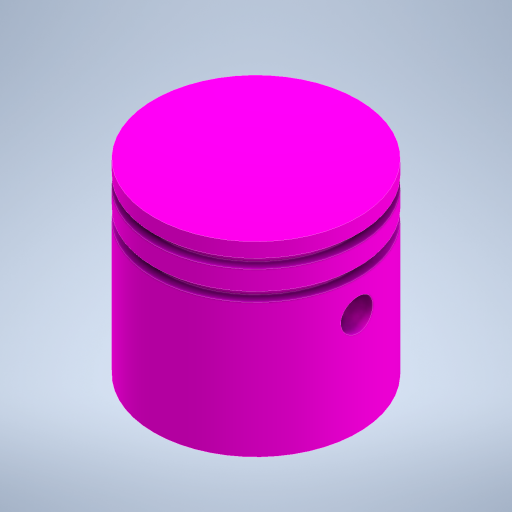
# Autodesk Inventor part: Piston_head
Saved by Autodesk Inventor 2024 (Build 280153000, 153)
## iProperties
Created: 2023-11-02
Part Number: Piston_head
Material: Ocel
Document SubType Name: Modeling
Designer: zak
Density: 7.85 g/cm^3
Appearance: Purpurová
Author: zak
Autodesk Inventor part; units mm, degrees
ref_plane "XZ Plane" through (0, 0, 0) normal (0, 1, 0) x (-1, 0, 0)
ref_plane "XY Plane" through (0, 0, 0) normal (0, 0, 1) x (1, 0, 0)
sketch "Náčrt3" plane through (0, 0, 0) normal (1, 0, 0) x (0, 1, 0)
  line L0 (0, 0) -> (0, 16)
  line L1 (0, 16) -> (21, 16)
  line L2 (21, 16) -> (21, 14.5)
  line L3 (21, 14.5) -> (22.5, 14.5)
  line L4 (22.5, 14.5) -> (22.5, 16)
  line L5 (22.5, 16) -> (25.5, 16)
  line L6 (25.5, 16) -> (25.5, 14.5)
  line L7 (25.5, 14.5) -> (27, 14.5)
  line L8 (27, 14.5) -> (27, 16)
  line L9 (27, 16) -> (29.2548, 16)
  line L10 (32, 0) -> (0, 0)
  arc A0 (32, 0) -> (29.2548, 16) centre (-16, 0) ccw
  dimension "d4" = 16
  dimension "d5" = 21
  dimension "d6" = 3
  dimension "d7" = 1.5
  dimension "d8" = 1.5
  dimension "d9" = 14.5
  dimension "d12" = 96
  dimension "d13" = 32
  constraints: 22 end point, 8 perpendicular, 2 collinear, 2 point on circle, 2 point on line, 1 centre point, 1 parallel, 1 vertical
  measures "d4" distance between parallel lines of L10 L1
  measures "d5" distance between parallel lines of L2 L0
  measures "d6" distance between parallel lines of L6 L4
  measures "d7" distance of L2.end L3.end
  measures "d8" distance of L6.end L7.end
  measures "d9" distance between parallel lines of L10 L3
  measures "d12" diameter of A0
  measures "d13" distance of L0.start L10.start
revolve "Rotace1" add sketch "Náčrt3" angle 360 about axis through (0, 32, 0) along (0, -1, 0)
sketch "Náčrt4" plane through (0, 0, 0) normal (1, 0, 0) x (0, 1, 0)
  line L0 (0, 16) -> (0, -16) projected
  line L1 (0, 13) -> (10, 13)
  line L2 (10, 13) -> (10, 10)
  line L3 (20.5263, 0) -> (0, 0)
  line L4 (10, 10) -> (24, 10)
  line L5 (24, 10) -> (24, 0)
  line L6 (24, 0) -> (20.5263, 0)
  line L7 (-6.4, 0) -> (38.4, 0) projected
  dimension "d14" = 10
  dimension "d15" = 13
  dimension "d16" = 10
  dimension "d17" = 24
  constraints: 12 end point, 3 perpendicular, 2 horizontal, 1 point on line, 1 vertical
  measures "d14" distance between parallel lines of L6 L4
  measures "d15" distance between parallel lines of L3 L1
  measures "d16" distance between parallel lines of L0 L2
  measures "d17" distance between parallel lines of L0 L5
revolve "Rotace2" cut sketch "Náčrt4" angle 360 about axis through (0, -10, 0) along (0, 1, 0)
fillet "Zaoblení1" radius 2 2 edges at (0, 10, -13) (0, 24, -10)
ref_plane "Pracovní rovina1" through (16, 0, 0) normal (1, 0, 0) x (0, 1, 0)
sketch "Náčrt5" plane through (16, 0, 0) normal (1, 0, 0) x (0, 1, 0)
  line L0 (-6.4, 0) -> (38.4, 0) projected
  line L1 (0, -22.4) -> (0, 22.4) projected
  point P0 (0, 0)
  point P1 (16, 0)
  dimension "d21" = 16
  constraints: 1 midpoint
  measures "d21" distance from line of L1 point (16, 0)
hole "Díra1" at (16, 16, 0) direction (-1, 0, 0) diameter 5 end through all
